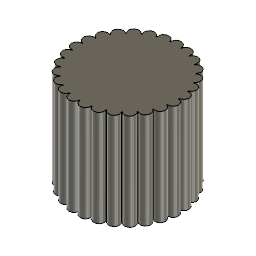
button_cap (Autodesk Fusion 360 design; units mm, degrees)
part number: 2026-01-18-21-26-09-885
Autodesk Fusion 360 part; units mm, degrees
sketch "Sketch1" plane through (0, 0, 0) normal (0, 0, 1) x (1, 0, 0)
  circle A0 centre (0, 0) radius 4.5
  dimension "d1" = 9
  constraint coincident A0.centre origin
  measures "d1" diameter of A0
extrude "Extrude1" add sketch "Sketch1" along normal blind 9
sketch "Sketch2" plane through (0, 0, 0) normal (0, 0, -1) x (1, 0, 0)
  circle A0 centre (0, 0) radius 4.5
  circle A1 centre (0, 0) radius 3.3
  dimension "d4" = 6.6
  constraint coincident A0.centre A1.centre
  measures "d4" diameter of A1
extrude "Extrude2" cut sketch "Sketch2" against normal blind 8 contours A1
chamfer "Chamfer1" distance 8 distance2 0.4 1 edges at (-3.0767, -1.1933, 8) measured on face at (3.2959, 0.1645, 5.3333)
sketch "Sketch3" plane through (0, 0, 9) normal (0, 0, 1) x (-1, 0, 0)
  circle A0 centre (0, 0) radius 4.5
  circle A1 centre (0, -4.5) radius 0.5
  circle A2 centre (1.0378, -4.3787) radius 0.5
  circle A3 centre (2.0196, -4.0213) radius 0.5
  circle A4 centre (2.8925, -3.4472) radius 0.5
  circle A5 centre (3.6096, -2.6872) radius 0.5
  circle A6 centre (4.132, -1.7824) radius 0.5
  circle A7 centre (4.4316, -0.7814) radius 0.5
  circle A8 centre (4.4924, 0.2617) radius 0.5
  circle A9 centre (4.311, 1.2906) radius 0.5
  circle A10 centre (3.8971, 2.25) radius 0.5
  circle A11 centre (3.2732, 3.0881) radius 0.5
  circle A12 centre (2.4728, 3.7597) radius 0.5
  circle A13 centre (1.5391, 4.2286) radius 0.5
  circle A14 centre (0.5224, 4.4696) radius 0.5
  circle A15 centre (-0.5224, 4.4696) radius 0.5
  circle A16 centre (-1.5391, 4.2286) radius 0.5
  circle A17 centre (-2.4728, 3.7597) radius 0.5
  circle A18 centre (-3.2732, 3.0881) radius 0.5
  circle A19 centre (-3.8971, 2.25) radius 0.5
  circle A20 centre (-4.311, 1.2906) radius 0.5
  circle A21 centre (-4.4924, 0.2617) radius 0.5
  circle A22 centre (-4.4316, -0.7814) radius 0.5
  circle A23 centre (-4.132, -1.7824) radius 0.5
  circle A24 centre (-3.6096, -2.6872) radius 0.5
  circle A25 centre (-2.8925, -3.4472) radius 0.5
  circle A26 centre (-2.0196, -4.0213) radius 0.5
  circle A27 centre (-1.0378, -4.3787) radius 0.5
  dimension "d9" = 1
  dimension "d11" = 360
  constraint coincident A0 A1.centre
  measures "d9" diameter of A1
extrude "Extrude3" add sketch "Sketch3" against normal blind 9 contours A0 A8 | A0 A9 | A0 A7 | A0 A10 | A0 A6 | A0 A11 | A0 A5 | A0 A12 | A0 A4 | A0 A13 | A0 A3 | A0 A14 | A0 A2 | A0 A15 | A0 A1 | A0 A16 | A0 A27 | A0 A17 | A0 A26 | A0 A18 | A0 A25 | A0 A19 | A0 A24 | A0 A20 | A0 A23 | A0 A21 | A0 A22 picked at (4.6266, 0.4296) picked at (4.4684, 1.3385) picked at (4.5947, -0.8041) picked at (4.0353, 2.3394) picked at (4.2812, -1.8519) picked at (3.3942, 3.1996) picked at (3.7345, -2.7944) picked at (2.5593, 3.8997) picked at (2.9972, -3.5743) picked at (1.5989, 4.382) picked at (2.0867, -4.1716) picked at (0.5394, 4.6333) picked at (1.0764, -4.5387) picked at (-0.5415, 4.6331) picked at (-0.0046, -4.6645) picked at (-1.5954, 4.3833) picked at (-1.0757, -4.5389) picked at (-2.5632, 3.8972) picked at (-2.0935, -4.1684) picked at (-3.3929, 3.201) picked at (-2.9984, -3.5733) picked at (-4.0397, 2.3323) picked at (-3.7416, -2.7855) picked at (-4.4686, 1.3378) picked at (-4.2831, -1.8476) picked at (-4.6567, 0.2712) picked at (-4.5937, -0.81)
